Autodesk Fusion 360 part; units mm, degrees
note: some values were not read from the file. Chosen so that the rebuilt part matches the saved one: which bodies a step acts on; which pieces of a blend or face edit are solid. Set by a fixed rule: which sketch regions a step uses; the direction of a hole.
(part 2 of 2)
  constraint tangent L118 A111
  constraint tangent L136 A111
  constraint equal A56 A111
  constraint tangent L131 A112
  constraint tangent L136 A112
  constraint equal A56 A112
  constraint tangent L124 A113
  constraint tangent L133 A113
  constraint equal A56 A113
  constraint tangent L117 A114
  constraint tangent L124 A114
  constraint equal A56 A114
  constraint tangent L139 A115
  constraint tangent L141 A115
  constraint equal A56 A115
  constraint tangent L141 A116
  constraint tangent L142 A116
  constraint equal A56 A116
  constraint tangent L142 A117
  constraint tangent L148 A117
  constraint equal A56 A117
  constraint tangent A115 A118
  constraint tangent L141 A118
  constraint equal A56 A118
  constraint tangent L139 A119
  constraint tangent L148 A119
  constraint equal A56 A119
  constraint tangent L147 A120
  constraint tangent L152 A120
  constraint equal A56 A120
  constraint tangent L150 A121
  constraint tangent L152 A121
  constraint equal A56 A121
  constraint tangent L144 A122
  constraint tangent L147 A122
  constraint equal A56 A122
  constraint tangent L144 A123
  constraint tangent L150 A123
  constraint equal A56 A123
  constraint tangent L140 A124
  constraint tangent L151 A124
  constraint equal A56 A124
  constraint tangent L145 A125
  constraint tangent L151 A125
  constraint equal A56 A125
  constraint tangent L140 A126
  constraint tangent L149 A126
  constraint equal A56 A126
  constraint tangent L145 A127
  constraint tangent L149 A127
  constraint equal A56 A127
  constraint tangent L271 A128
  constraint tangent L272 A128
  constraint equal A56 A128
  constraint coincident P21 L272
  constraint coincident P21 L273
  constraint tangent L272 A129
  constraint tangent L273 A129
  constraint equal A56 A129
  constraint coincident P19 L270
  constraint coincident P19 L273
  constraint tangent L270 A130
  constraint tangent L273 A130
  constraint equal A56 A130
  constraint coincident P20 L270
  constraint coincident P20 L271
  constraint tangent L270 A131
  constraint tangent L271 A131
  constraint equal A56 A131
  constraint coincident L128.end L130
  constraint coincident L128.end L112
  constraint tangent L130 A132
  constraint tangent L112 A132
  constraint coincident P18 L267
  constraint coincident P18 L268
  constraint tangent L267 A133
  constraint tangent L268 A133
  constraint tangent L266 A134
  constraint tangent L267 A134
  constraint equal A133 A134
  constraint tangent L265 A135
  constraint tangent L266 A135
  constraint equal A133 A135
  constraint coincident P17 L265
  constraint coincident P17 L268
  constraint tangent L265 A136
  constraint tangent L268 A136
  constraint equal A133 A136
  constraint tangent L249 A137
  constraint tangent L259 A137
  constraint equal A133 A137
  constraint tangent L253 A138
  constraint tangent L259 A138
  constraint equal A133 A138
  constraint tangent L253 A139
  constraint tangent L254 A139
  constraint equal A133 A139
  constraint tangent L249 A140
  constraint tangent L254 A140
  constraint equal A133 A140
  constraint tangent L255 A141
  constraint tangent L260 A141
  constraint equal A133 A141
  constraint tangent L257 A142
  constraint tangent L260 A142
  constraint equal A133 A142
  constraint tangent L251 A143
  constraint tangent L257 A143
  constraint equal A133 A143
  constraint tangent L251 A144
  constraint tangent L255 A144
  constraint equal A133 A144
  constraint tangent L256 A145
  constraint tangent L263 A145
  constraint equal A133 A145
  constraint tangent L263 A146
  constraint tangent L264 A146
  constraint equal A133 A146
  constraint tangent L252 A147
  constraint tangent L264 A147
  constraint equal A133 A147
  constraint tangent L252 A148
  constraint tangent L256 A148
  constraint equal A133 A148
  constraint tangent L250 A149
  constraint tangent L261 A149
  constraint equal A133 A149
  constraint tangent L261 A150
  constraint tangent L262 A150
  constraint equal A133 A150
  constraint tangent L250 A151
  constraint tangent L258 A151
  constraint equal A133 A151
  constraint tangent L258 A152
  constraint tangent L262 A152
  constraint equal A133 A152
  constraint tangent L242 A153
  constraint tangent L246 A153
  constraint equal A133 A153
  constraint tangent L229 A154
  constraint tangent L242 A154
  constraint equal A133 A154
  constraint tangent L229 A155
  constraint tangent L245 A155
  constraint equal A133 A155
  constraint tangent L245 A156
  constraint tangent L246 A156
  constraint equal A133 A156
  constraint tangent L235 A157
  constraint tangent L248 A157
  constraint equal A133 A157
  constraint tangent L248 A158
  constraint tangent L247 A158
  constraint equal A133 A158
  constraint tangent L240 A159
  constraint tangent L247 A159
  constraint equal A133 A159
  constraint tangent L235 A160
  constraint tangent L240 A160
  constraint equal A133 A160
  constraint tangent L241 A161
  constraint tangent L244 A161
  constraint equal A133 A161
  constraint tangent L234 A162
  constraint tangent L241 A162
  constraint equal A133 A162
  constraint tangent L238 A163
  constraint tangent L244 A163
  constraint equal A133 A163
  constraint tangent L234 A164
  constraint tangent L238 A164
  constraint equal A133 A164
  constraint tangent L236 A165
  constraint tangent L243 A165
  constraint equal A133 A165
  constraint tangent L236 A166
  constraint tangent L237 A166
  constraint equal A133 A166
  constraint tangent L225 A167
  constraint tangent L243 A167
  constraint equal A133 A167
  constraint tangent L225 A168
  constraint tangent L237 A168
  constraint equal A133 A168
  constraint tangent L201 A169
  constraint tangent L219 A169
  constraint equal A133 A169
  constraint tangent L201 A170
  constraint tangent L213 A170
  constraint equal A133 A170
  constraint tangent L212 A171
  constraint tangent L219 A171
  constraint equal A133 A171
  constraint tangent L212 A172
  constraint tangent L213 A172
  constraint equal A133 A172
  constraint tangent L214 A173
  constraint tangent L220 A173
  constraint equal A133 A173
  constraint tangent L210 A174
  constraint tangent L214 A174
  constraint equal A133 A174
  constraint tangent L217 A175
  constraint tangent L220 A175
  constraint equal A133 A175
  constraint tangent L210 A176
  constraint tangent L217 A176
  constraint equal A133 A176
  constraint tangent L216 A177
  constraint tangent L223 A177
  constraint equal A133 A177
  constraint tangent L211 A178
  constraint tangent L216 A178
  constraint equal A133 A178
  constraint tangent L223 A179
  constraint tangent L224 A179
  constraint equal A133 A179
  constraint tangent L211 A180
  constraint tangent L224 A180
  constraint equal A133 A180
  constraint tangent L205 A181
  constraint tangent L221 A181
  constraint equal A133 A181
  constraint tangent L221 A182
  constraint tangent L222 A182
  constraint equal A133 A182
  constraint tangent L205 A183
  constraint tangent L218 A183
  constraint equal A133 A183
  constraint tangent L218 A184
  constraint tangent L222 A184
  constraint equal A133 A184
  constraint tangent L227 A185
  constraint tangent L230 A185
  constraint equal A133 A185
  constraint tangent L227 A186
  constraint tangent L228 A186
  constraint equal A133 A186
  constraint tangent L230 A187
  constraint tangent L231 A187
  constraint equal A133 A187
  constraint tangent L228 A188
  constraint tangent L231 A188
  constraint equal A133 A188
  constraint tangent L226 A189
  constraint tangent L233 A189
  constraint equal A133 A189
  constraint tangent L233 A190
  constraint tangent L239 A190
  constraint equal A133 A190
  constraint tangent L226 A191
  constraint tangent L232 A191
  constraint equal A133 A191
  constraint tangent L232 A192
  constraint tangent L239 A192
  constraint equal A133 A192
  constraint tangent L203 A193
  constraint tangent L206 A193
  constraint equal A133 A193
  constraint tangent L206 A194
  constraint tangent L207 A194
  constraint equal A133 A194
  constraint tangent L204 A195
  constraint tangent L207 A195
  constraint equal A133 A195
  constraint tangent L203 A196
  constraint tangent L204 A196
  constraint equal A133 A196
  constraint tangent L202 A197
  constraint tangent L209 A197
  constraint equal A133 A197
  constraint tangent L202 A198
  constraint tangent L208 A198
  constraint equal A133 A198
  constraint tangent L208 A199
  constraint tangent L215 A199
  constraint equal A133 A199
  constraint tangent L209 A200
  constraint tangent L215 A200
  constraint equal A133 A200
  constraint tangent L181 A201
  constraint tangent L190 A201
  constraint equal A133 A201
  constraint tangent L190 A202
  constraint tangent L197 A202
  constraint equal A133 A202
  constraint tangent L178 A203
  constraint tangent L181 A203
  constraint equal A133 A203
  constraint tangent L178 A204
  constraint tangent L197 A204
  constraint equal A133 A204
  constraint tangent L177 A205
  constraint tangent L198 A205
  constraint equal A133 A205
  constraint tangent L180 A206
  constraint tangent L198 A206
  constraint equal A133 A206
  constraint tangent L180 A207
  constraint tangent L193 A207
  constraint equal A133 A207
  constraint tangent L177 A208
  constraint tangent L193 A208
  constraint equal A133 A208
  constraint tangent L192 A209
  constraint tangent L196 A209
  constraint equal A133 A209
  constraint tangent L179 A210
  constraint tangent L192 A210
  constraint equal A133 A210
  constraint tangent L179 A211
  constraint tangent L199 A211
  constraint equal A133 A211
  constraint tangent L196 A212
  constraint tangent L199 A212
  constraint equal A133 A212
  constraint tangent L185 A213
  constraint tangent L194 A213
  constraint equal A133 A213
  constraint tangent L185 A214
  constraint tangent L186 A214
  constraint equal A133 A214
  constraint tangent L186 A215
  constraint tangent L188 A215
  constraint equal A133 A215
  constraint tangent L188 A216
  constraint tangent L194 A216
  constraint equal A133 A216
  constraint tangent L166 A217
  constraint tangent L168 A217
  constraint equal A133 A217
  constraint tangent L167 A218
  constraint tangent L168 A218
  constraint equal A133 A218
  constraint tangent L165 A219
  constraint tangent L167 A219
  constraint equal A133 A219
  constraint tangent L165 A220
  constraint tangent L166 A220
  constraint equal A133 A220
  constraint tangent L163 A221
  constraint tangent L164 A221
  constraint equal A133 A221
  constraint tangent L161 A222
  constraint tangent L163 A222
  constraint equal A133 A222
  constraint tangent L162 A223
  constraint tangent L164 A223
  constraint equal A133 A223
  constraint tangent L161 A224
  constraint tangent L162 A224
  constraint equal A133 A224
  constraint tangent L159 A225
  constraint tangent L160 A225
  constraint equal A133 A225
  constraint tangent L157 A226
  constraint tangent L159 A226
  constraint equal A133 A226
  constraint tangent L158 A227
  constraint tangent L160 A227
  constraint equal A133 A227
  constraint tangent L157 A228
  constraint tangent L158 A228
  constraint equal A133 A228
  constraint tangent L154 A229
  constraint tangent L155 A229
  constraint equal A133 A229
  constraint tangent L153 A230
  constraint tangent L154 A230
  constraint equal A133 A230
  constraint tangent L155 A231
  constraint tangent L156 A231
  constraint equal A133 A231
  constraint tangent L153 A232
  constraint tangent L156 A232
  constraint equal A133 A232
  constraint tangent L170 A233
  constraint tangent L172 A233
  constraint equal A133 A233
  constraint tangent L171 A234
  constraint tangent L172 A234
  constraint equal A133 A234
  constraint tangent L169 A235
  constraint tangent L171 A235
  constraint equal A133 A235
  constraint tangent L169 A236
  constraint tangent L170 A236
  constraint equal A133 A236
  constraint tangent L173 A237
  constraint tangent L174 A237
  constraint equal A133 A237
  constraint tangent L174 A238
  constraint tangent L176 A238
  constraint equal A133 A238
  constraint tangent L175 A239
  constraint tangent L176 A239
  constraint equal A133 A239
  constraint tangent L173 A240
  constraint tangent L175 A240
  constraint equal A133 A240
  constraint tangent L184 A241
  constraint tangent L187 A241
  constraint equal A133 A241
  constraint tangent L182 A242
  constraint tangent L184 A242
  constraint equal A133 A242
  constraint tangent L182 A243
  constraint tangent L183 A243
  constraint equal A133 A243
  constraint tangent L183 A244
  constraint tangent L187 A244
  constraint equal A133 A244
  constraint tangent L189 A245
  constraint tangent L200 A245
  constraint equal A133 A245
  constraint tangent L189 A246
  constraint tangent L191 A246
  constraint equal A133 A246
  constraint tangent L191 A247
  constraint tangent L195 A247
  constraint equal A133 A247
  constraint tangent L195 A248
  constraint tangent L200 A248
  constraint equal A133 A248
  measures "d1" distance of L6.start L0.start
  measures "d2" distance of L0.start L0.end
  measures "d3" distance of L0.end L1.end
  measures "d7" distance of L4.end L5.end
  measures "d11" distance of L7.start L7.end
  measures "d12" distance of L7.end L8.end
  measures "d13" distance of L8.end L9.end
  measures "d15" distance of L10.end L11.end
  measures "d18" distance of L12.end L13.end
  measures "d87" distance of P17 P18
  measures "d90" distance of L13.end L269.end
  measures "d92" distance of P19 P21
  measures "d93" distance of P19 P20
  measures "d94" radius of A0
  measures "d95" radius of A16
  measures "d96" radius of A54
  measures "d97" radius of A55
  measures "d98" radius of A56
  measures "d99" radius of A132
  measures "d100" radius of A133
  measures "d105" distance of L11.end P22
extrude "Extrude1" add sketch "Sketch1" along normal blind 4 contours L0 L1 L2 L3 L4 L5 L6 L15 | L7 L8 L9 L10 L11 L12 L13 L14 L32 L269 | L16 L17 L18 L19 L20 L21 L22 L23 A8 A9 A10 A11 A12 A13 A14 A15 | L24 L25 L26 L27 L28 L29 L30 L31 A0 A1 A2 A3 A4 A5 A6 A7 makes body 1 at (38.1433, 0, -12.1134) makes body 2 at (-23.9522, 0, -12.611)
extrude "Extrude2" add sketch "Sketch1" against normal blind 1 contours L16 L17 L18 L19 L20 L21 L22 L23 A8 A9 A10 A11 A12 A13 A14 A15 | L24 L25 L26 L27 L28 L29 L30 L31 A0 A1 A2 A3 A4 A5 A6 A7 bodies 1 2
hole "Hole1" at (-123.1355, 0, 35.5) at (-18.6355, 0, 47) at (-125.6355, 0, 54.5) at (-9.1355, 0, 54.5) at (-9.1355, 0, -49) at (-161.6355, 0, -49) at (-161.6355, 0, 36.5) at (-155.1355, 0, -42) at (-15.3855, 0, -43.25) at (29.5, 0, -43) at (23.0255, 0, -48.5253) at (170.75, 0, -42) at (177.25, 0, -48.5) at (177.25, 0, 37) at (140.75, 0, 55) at (140.2499, 0, 35.0254) at (22, 0, 55) at (31.9999, 0, 47.1754) direction (0, 1, 0) diameter 2.1 end through all bodies 2 1
move_body "Move1" bodies 1 2 to x (1, 0, 0) y (0, 1, 0) z (0, 0, 1) at (0, 0, -140)
extrude "Extrude3" add sketch "Sketch1" along normal blind 8 separate body contours L0 L1 L2 L3 L4 L5 L6 L15 | L7 L8 L9 L10 L11 L12 L13 L14 L32 L269 | L16 L17 L18 L19 L20 L21 L22 L23 A8 A9 A10 A11 A12 A13 A14 A15 | L24 L25 L26 L27 L28 L29 L30 L31 A0 A1 A2 A3 A4 A5 A6 A7 | L34 L35 L36 L37 L38 A16 A17 A18 A54 | L39 L40 L41 L42 A19 A20 A21 A22 | L43 L44 L45 L46 A23 A24 A25 A26 | L47 L48 L49 L50 A27 A28 A29 A30 | L51 L52 L53 L54 A46 A47 A48 A49 | L55 L56 L57 L58 A84 A85 A86 A87 | L59 L64 L81 L84 A80 A81 A82 A83 | L60 L63 L73 L74 A39 A40 A41 A42 | L61 L62 L70 L71 L75 A43 A44 A45 A55 | L65 L66 L76 L79 A35 A36 A37 A38 | L67 L68 L78 L80 A31 A32 A33 A34 | L72 L77 L82 L83 A50 A51 A52 A53 | L85 L98 L104 L109 A60 A61 A62 A63 | L86 L95 L100 L101 A72 A73 A74 A75 | L87 L88 L96 L97 A68 A69 A70 A71 | L89 L90 L93 L94 A76 A77 A78 A79 | L91 L92 L99 L106 L110 A56 A57 A58 A59 | L102 L103 L105 L107 A64 A65 A66 A67 | L111 L113 L114 L132 A91 A92 A93 A94 | L112 L116 L128 L129 L130 A88 A89 A90 A132 | L115 L119 L121 L126 A99 A100 A101 A102 | L117 L124 L127 L133 A103 A104 A113 A114 | L118 L123 L131 L136 A105 A106 A111 A112 | L120 L125 L134 L135 A107 A108 A109 A110 | L137 L138 L143 L146 A95 A96 A97 A98 | L139 L141 L142 L148 A115 A116 A117 A118 A119 | L140 L145 L149 L151 A124 A125 A126 A127 | L144 L147 L150 L152 A120 A121 A122 A123 | L153 L154 L155 L156 A229 A230 A231 A232 | L157 L158 L159 L160 A225 A226 A227 A228 | L161 L162 L163 L164 A221 A222 A223 A224 | L165 L166 L167 L168 A217 A218 A219 A220 | L169 L170 L171 L172 A233 A234 A235 A236 | L173 L174 L175 L176 A237 A238 A239 A240 | L177 L180 L193 L198 A205 A206 A207 A208 | L178 L181 L190 L197 A201 A202 A203 A204 | L179 L192 L196 L199 A209 A210 A211 A212 | L182 L183 L184 L187 A241 A242 A243 A244 | L185 L186 L188 L194 A213 A214 A215 A216 | L189 L191 L195 L200 A245 A246 A247 A248 | L201 L212 L213 L219 A169 A170 A171 A172 | L202 L208 L209 L215 A197 A198 A199 A200 | L203 L204 L206 L207 A193 A194 A195 A196 | L205 L218 L221 L222 A181 A182 A183 A184 | L210 L214 L217 L220 A173 A174 A175 A176 | L211 L216 L223 L224 A177 A178 A179 A180 | L225 L236 L237 L243 A165 A166 A167 A168 | L226 L232 L233 L239 A189 A190 A191 A192 | L227 L228 L230 L231 A185 A186 A187 A188 | L229 L242 L245 L246 A153 A154 A155 A156 | L234 L238 L241 L244 A161 A162 A163 A164 | L235 L240 L247 L248 A157 A158 A159 A160 | L249 L253 L254 L259 A137 A138 A139 A140 | L250 L258 L261 L262 A149 A150 A151 A152 | L251 L255 L257 L260 A141 A142 A143 A144 | L252 L256 L263 L264 A145 A146 A147 A148 | L265 L266 L267 L268 A133 A134 A135 A136 | L270 L271 L272 L273 A128 A129 A130 A131 makes body 3 at (-99.9688, 0, -18.744) makes body 4 at (114.8434, 0, -18.244)
extrude "Extrude4" add sketch "Sketch1" along normal blind 13 separate body contours L16 L17 L18 L19 L20 L21 L22 L23 A8 A9 A10 A11 A12 A13 A14 A15 | L24 L25 L26 L27 L28 L29 L30 L31 A0 A1 A2 A3 A4 A5 A6 A7 makes body 5 at (-109.9688, 0, -49.8333) makes body 6 at (125.0101, 0, -49.3333)
combine "Combine1" operation add target body 3 tool bodies 5
combine "Combine2" operation add target body 6 tool bodies 4
sketch "Sketch2" plane through (0, 0, 0) normal (0, 1, 0) x (1, 0, 0)
  line L0 (-145, 32.4457) -> (-45, 32.4457)
  line L1 (-45, 32.4457) -> (-45, -27.5543)
  line L2 (-45, -27.5543) -> (-145, -27.5543)
  line L3 (-145, -27.5543) -> (-145, 32.4457)
  line L4 (60, 32.4457) -> (160, 32.4457)
  line L5 (160, -27.5543) -> (60, -27.5543)
  line L6 (160, 32.4457) -> (160, -27.5543)
  line L7 (60, -27.5543) -> (60, 32.4457)
  line L8 (-35, 40) -> (-15, 40)
  line L9 (-15, 40) -> (-15, 10)
  line L10 (-15, 10) -> (-35, 10)
  line L11 (-35, 10) -> (-35, 40)
  circle A0 centre (-30, 17.5) radius 2
  circle A1 centre (-20, 17.5) radius 2
  circle A2 centre (-20, 32.5) radius 2
  circle A3 centre (-30, 32.5) radius 2
  line L12 (-45.5, 25) -> (-34.5, 25)
  line L13 (-34.5, 25) -> (-34.5, 22)
  line L14 (-34.5, 22) -> (-45.5, 22)
  line L15 (-45.5, 22) -> (-45.5, 25)
  line L16 (60.5, 25) -> (49.5, 25)
  line L17 (49.5, 22) -> (60.5, 22)
  line L18 (49.5, 25) -> (49.5, 22)
  line L19 (50, 10) -> (50, 40)
  line L20 (60.5, 22) -> (60.5, 25)
  circle A4 centre (45, 32.5) radius 2
  circle A5 centre (35, 32.5) radius 2
  circle A6 centre (35, 17.5) radius 2
  circle A7 centre (45, 17.5) radius 2
  line L21 (30, 40) -> (30, 10)
  line L22 (30, 10) -> (50, 10)
  line L23 (50, 40) -> (30, 40)
  line L24 (-30, -5) -> (-32.5, -9.3301)
  line L25 (-32.5, -9.3301) -> (-30, -13.6603)
  line L26 (-30, -13.6603) -> (-25, -13.6603)
  line L27 (-25, -13.6603) -> (-22.5, -9.3301)
  line L28 (-22.5, -9.3301) -> (-25, -5)
  line L29 (-25, -5) -> (-30, -5)
  line L30 (-16, -8.6603) -> (-13.5, -4.3301)
  line L31 (-21, -8.6603) -> (-16, -8.6603)
  line L32 (-16, 0) -> (-21, 0)
  line L33 (-13.5, -4.3301) -> (-16, 0)
  line L34 (-23.5, -4.3301) -> (-21, -8.6603)
  line L35 (-21, 0) -> (-23.5, -4.3301)
  line L36 (-16, -18.6603) -> (-13.5, -14.3301)
  line L37 (-21, -18.6603) -> (-16, -18.6603)
  line L38 (-16, -10) -> (-21, -10)
  line L39 (-13.5, -14.3301) -> (-16, -10)
  line L40 (-23.5, -14.3301) -> (-21, -18.6603)
  line L41 (-21, -10) -> (-23.5, -14.3301)
  line L42 (-25, -3.6603) -> (-22.5, 0.6699)
  line L43 (-30, -3.6603) -> (-25, -3.6603)
  line L44 (-25, 5) -> (-30, 5)
  line L45 (-22.5, 0.6699) -> (-25, 5)
  line L46 (-32.5, 0.6699) -> (-30, -3.6603)
  line L47 (-30, 5) -> (-32.5, 0.6699)
  line L48 (-25, -23.6603) -> (-22.5, -19.3301)
  line L49 (-30, -23.6603) -> (-25, -23.6603)
  line L50 (-25, -15) -> (-30, -15)
  line L51 (-22.5, -19.3301) -> (-25, -15)
  line L52 (-32.5, -19.3301) -> (-30, -23.6603)
  line L53 (-30, -15) -> (-32.5, -19.3301)
  line L54 (-16, 1.3397) -> (-13.5, 5.6699)
  line L55 (-21, 1.3397) -> (-16, 1.3397)
  line L56 (-16, 10) -> (-21, 10)
  line L57 (-13.5, 5.6699) -> (-16, 10)
  line L58 (-23.5, 5.6699) -> (-21, 1.3397)
  line L59 (-21, 10) -> (-23.5, 5.6699)
  line L60 (-34, -33.6603) -> (-31.5, -29.3301)
  line L61 (-39, -33.6603) -> (-34, -33.6603)
  line L62 (-34, -25) -> (-39, -25)
  line L63 (-31.5, -29.3301) -> (-34, -25)
  line L64 (-41.5, -29.3301) -> (-39, -33.6603)
  line L65 (-39, -25) -> (-41.5, -29.3301)
  line L66 (-25, -13.6603) -> (-22.5, -9.3301)
  line L67 (-30, -13.6603) -> (-25, -13.6603)
  line L68 (-25, -5) -> (-30, -5)
  line L69 (-22.5, -9.3301) -> (-25, -5)
  line L70 (-32.5, -9.3301) -> (-30, -13.6603)
  line L71 (-30, -5) -> (-32.5, -9.3301)
  line L72 (39, -14.3301) -> (36.5, -18.6603)
  line L73 (39, 5.6699) -> (36.5, 1.3397)
  line L74 (36.5, -18.6603) -> (31.5, -18.6603)
  line L75 (40.5, -5) -> (45.5, -5)
  line L76 (45.5, 5) -> (48, 0.6699)
  line L77 (36.5, 10) -> (39, 5.6699)
  line L78 (36.5, 0) -> (39, -4.3301)
  line L79 (31.5, -8.6603) -> (29, -4.3301)
  line L80 (29, 5.6699) -> (31.5, 10)
  line L81 (38, 0.6699) -> (40.5, 5)
  line L82 (38, -9.3301) -> (40.5, -5)
  line L83 (45.5, -5) -> (48, -9.3301)
  line L84 (29, -4.3301) -> (31.5, 0)
  line L85 (40.5, -23.6603) -> (38, -19.3301)
  line L86 (48, -9.3301) -> (45.5, -13.6603)
  line L87 (29, -14.3301) -> (31.5, -10)
  line L88 (48, -19.3301) -> (45.5, -23.6603)
  line L89 (48, -9.3301) -> (45.5, -13.6603)
  line L90 (45.5, -13.6603) -> (40.5, -13.6603)
  line L91 (40.5, -13.6603) -> (38, -9.3301)
  line L92 (40.5, -3.6603) -> (38, 0.6699)
  line L93 (40.5, 5) -> (45.5, 5)
  line L94 (31.5, 1.3397) -> (29, 5.6699)
  line L95 (36.5, 1.3397) -> (31.5, 1.3397)
  line L96 (31.5, 0) -> (36.5, 0)
  line L97 (45.5, -3.6603) -> (40.5, -3.6603)
  line L98 (48, 0.6699) -> (45.5, -3.6603)
  line L99 (40.5, -5) -> (45.5, -5)
  line L100 (31.5, 10) -> (36.5, 10)
  line L101 (39, -4.3301) -> (36.5, -8.6603)
  line L102 (38, -9.3301) -> (40.5, -5)
  line L103 (49.5, -25) -> (54.5, -25)
  line L104 (30.5, 10) -> (50.5, 10)
  line L105 (45.5, -5) -> (48, -9.3301)
  line L106 (36.5, -10) -> (39, -14.3301)
  line L107 (31.5, -18.6603) -> (29, -14.3301)
  line L108 (40.5, -15) -> (45.5, -15)
  line L109 (45.5, -23.6603) -> (40.5, -23.6603)
  line L110 (38, -19.3301) -> (40.5, -15)
  line L111 (45.5, -13.6603) -> (40.5, -13.6603)
  line L112 (31.5, -10) -> (36.5, -10)
  line L113 (40.5, -13.6603) -> (38, -9.3301)
  line L114 (36.5, -8.6603) -> (31.5, -8.6603)
  line L115 (45.5, -15) -> (48, -19.3301)
  line L116 (57, -29.3301) -> (54.5, -33.6603)
  line L117 (47, -29.3301) -> (49.5, -25)
  line L118 (54.5, -33.6603) -> (49.5, -33.6603)
  line L119 (49.5, -33.6603) -> (47, -29.3301)
  line L120 (54.5, -25) -> (57, -29.3301)
  line L121 (-2.7, 45) -> (0.1, 45)
  line L122 (0.4, 44.7) -> (0.4, 36.1)
  line L123 (0.1, 35.8) -> (-2.7, 35.8)
  line L124 (-3, 36.1) -> (-3, 44.7)
  arc A8 (0.4, 44.7) -> (0.1, 45) centre (0.1, 44.7) ccw
  arc A9 (-2.7, 45) -> (-3, 44.7) centre (-2.7, 44.7) ccw
  arc A10 (-3, 36.1) -> (-2.7, 35.8) centre (-2.7, 36.1) ccw
  arc A11 (0.1, 35.8) -> (0.4, 36.1) centre (0.1, 36.1) ccw
  line L125 (-3.5, 34) -> (2.7, 34)
  line L126 (3, 33.7) -> (3, 21.5)
  line L127 (2.7, 21.2) -> (-3.5, 21.2)
  line L128 (-3.8, 21.5) -> (-3.8, 33.7)
  arc A12 (-3.5, 34) -> (-3.8, 33.7) centre (-3.5, 33.7) ccw
  arc A13 (3, 33.7) -> (2.7, 34) centre (2.7, 33.7) ccw
  arc A14 (2.7, 21.2) -> (3, 21.5) centre (2.7, 21.5) ccw
  arc A15 (-3.8, 21.5) -> (-3.5, 21.2) centre (-3.5, 21.5) ccw
  point P0 (-27.5, -9.3301)
  point P1 (-18.5, -4.3301)
  point P2 (-18.5, -14.3301)
  point P3 (-27.5, 0.6699)
  point P4 (-27.5, -19.3301)
  point P5 (-18.5, 5.6699)
  point P6 (-36.5, -29.3301)
  point P7 (-27.5, -9.3301)
  point P8 (15.5, 0)
  point P9 (43, -9.3301)
  point P10 (52, -29.3301)
  point P11 (34, -4.3301)
  point P12 (43, -9.3301)
  point P13 (34, -14.3301)
  point P14 (43, -19.3301)
  point P15 (43, 0.6699)
  point P16 (34, 5.6699)
  point P17 (-3, 45)
  point P18 (0.4, 45)
  point P19 (-3, 35.8)
  point P20 (-3.8, 34)
  point P21 (3, 21.2)
  point P22 (-3.8, 21.2)
  dimension "d138" = 3.4
  dimension "d139" = 9.2
  dimension "d140" = 0.3
  dimension "d141" = 6.8
  dimension "d142" = 12.8
  dimension "d143" = 0.3
  constraint horizontal L0
  constraint vertical L1
  constraint horizontal L2
  constraint vertical L3
  constraint horizontal L4
  constraint vertical L6
  constraint horizontal L5
  constraint vertical L7
  constraint horizontal L8
  constraint vertical L9
  constraint horizontal L10
  constraint vertical L11
  constraint horizontal L12
  constraint perpendicular L12 L13
  constraint perpendicular L1 L14
  constraint perpendicular L12 L15
  constraint perpendicular L16 L18
  constraint perpendicular L16 L20
  constraint horizontal L121
  constraint vertical L122
  constraint horizontal L123
  constraint vertical L124
  constraint coincident P18 L121
  constraint coincident P18 L122
  constraint tangent L121 A8
  constraint tangent L122 A8
  constraint coincident P17 L121
  constraint coincident P17 L124
  constraint tangent L121 A9
  constraint tangent L124 A9
  constraint equal A8 A9
  constraint coincident P19 L123
  constraint coincident P19 L124
  constraint tangent L123 A10
  constraint tangent L124 A10
  constraint equal A8 A10
  constraint tangent L122 A11
  constraint tangent L123 A11
  constraint equal A8 A11
  constraint horizontal L125
  constraint vertical L126
  constraint horizontal L127
  constraint vertical L128
  constraint coincident P20 L125
  constraint coincident P20 L128
  constraint tangent L125 A12
  constraint tangent L128 A12
  constraint tangent L125 A13
  constraint tangent L126 A13
  constraint equal A12 A13
  constraint coincident P21 L126
  constraint coincident P21 L127
  constraint tangent L126 A14
  constraint tangent L127 A14
  constraint equal A12 A14
  constraint coincident P22 L127
  constraint coincident P22 L128
  constraint tangent L127 A15
  constraint tangent L128 A15
  constraint equal A12 A15
  measures "d138" distance of P17 P18
  measures "d139" distance of P17 P19
  measures "d140" radius of A8
  measures "d141" distance of P21 P22
  measures "d142" distance of P20 P22
  measures "d143" radius of A12
extrude "Extrude5" add sketch "Sketch2" along normal blind 4.5 separate body contours L0 L1 L2 L3 L12 L14 L15 | L1 L12 L14 L15 | L4 L5 L6 L7 L16 L17 L20 | L7 L16 L17 L20 makes body 7 at (-111.6667, 0, -12.4457) makes body 8 at (93.3333, 0, -12.4457)
move_body "Move2" bodies 7 8 to x (1, 0, 0) y (0, 1, 0) z (0, 0, 1) at (0, 4, 0)
combine "Combine3" operation cut target body 3 tool bodies 7
combine "Combine4" operation cut target body 6 tool bodies 8
chamfer "Chamfer1" distance 2 angle 45 8 edges at (110, 8, -32.4457) (110, 4, -32.4457) (60, 8, -2.4457) (160, 8, -2.4457) (160, 4, -2.4457) (110, 8, 27.5543) (110, 4, 27.5543) (60, 4, -2.4457) on bodies 6
chamfer "Chamfer2" distance 2 angle 45 8 edges at (-145, 4, -2.4457) (-145, 8, -2.4457) (-95, 8, -32.4457) (-95, 4, -32.4457) (-95, 8, 27.5543) (-45, 8, -2.4457) (-45, 4, -2.4457) (-95, 4, 27.5543) on bodies 3
extrude "Extrude6" add sketch "Sketch2" along normal blind 3 separate body contours L7 L16 L17 L20 | L7 L16 L17 L19 | L16 L17 L18 L19 | L16 L17 L18 L19 L21 L22 L23 L100 L104 | A4 | A5 | A6 | A7 makes body 9
move_body "Move3" bodies 9 to x (1, 0, 0) y (0, 1, 0) z (0, 0, 1) at (0, 5, -6)
combine "Combine5" operation cut target body 6 tool bodies 9
chamfer "Chamfer3" distance 0.5 angle 45 16 edges at (54, 8, -28) (54, 8, -31) (59.25, 6.75, -28) (59.25, 6.75, -31) (50, 6.5, -28) (50, 5, -22) (50, 8, -22) (50, 6.5, -31) (50, 8, -38.5) (50, 5, -38.5) (40, 5, -16) (40, 8, -16) (30, 8, -31) (30, 5, -31) (30, 6.5, -16) (50, 6.5, -16) on bodies 6
extrude "Extrude7" add sketch "Sketch2" along normal blind 3 separate body contours L1 L11 L12 L14 | L1 L12 L14 L15 | L11 L12 L13 L14 | L8 L9 L10 L11 L12 L13 L14 L56 | A0 | A1 | A2 | A3 makes body 10
move_body "Move4" bodies 10 to x (1, 0, 0) y (0, 1, 0) z (0, 0, 1) at (0, 0, -6.5)
move_body "Move5" bodies 10 to x (1, 0, 0) y (0, 1, 0) z (0, 0, 1) at (0, 5, 0)
combine "Combine6" operation cut target body 3 tool bodies 10
chamfer "Chamfer4" distance 0.5 angle 45 14 edges at (-15, 8, -31.5) (-15, 5, -31.5) (-35, 8, -39) (-39, 8, -31.5) (-39, 8, -28.5) (-35, 8, -22.5) (-25, 8, -16.5) (-35, 5, -22.5) (-25, 5, -16.5) (-35, 6.5, -16.5) (-35, 6.5, -28.5) (-35, 6.5, -31.5) (-35, 5, -39) (-15, 6.5, -16.5) on bodies 3
chamfer "Chamfer5" distance 0.5 angle 45 2 edges at (-35, 6.5, -46.5) (-45.5, 5.5, -30) on bodies 3
chamfer "Chamfer6" distance 0.5 angle 45 1 edges at (60.5, 5.5, -29.5) on bodies 6
chamfer "Chamfer7" distance 0.5 angle 45 8 edges at (25, 13, 3.25) (100.125, 13, -46) (81.375, 13, 52.5) (138.25, 13, 47.25) (144, 13, 42) (149.75, 13, 38.25) (162.25, 13, 34.5) (174.75, 13, -5.75) on bodies 6
chamfer "Chamfer8" distance 0.5 angle 45 8 edges at (-159.1355, 13, -6.25) (-85.3855, 13, -46.5) (-146.8855, 13, 34) (-134.6355, 13, 37.75) (-128.8855, 13, 41.5) (-123.1355, 13, 46.75) (-67.3855, 13, 52) (-11.6355, 13, 2.75) on bodies 3
extrude "Extrude8" add sketch "Sketch2" along normal blind 2 separate body contours A0 | A1 | A2 | A3 | A4 | A5 | A6 | A7 makes body 11 at (35.5417, 1.3333, -19.4252) makes body 12 at (-18.0025, 1.3333, -17.4003) makes body 13 at (-21.9382, 0.6667, -32.9935) makes body 14 at (45.5417, 1.3333, -19.4252) makes body 15 at (35.0499, 1.3333, -34.4994) makes body 16 at (-28.0025, 1.3333, -17.4003) makes body 17 at (-31.9901, 1.3333, -32.3009) makes body 18 at (44.363, 1.3333, -30.6041)
move_body "Move6" bodies 12 13 16 17 to x (1, 0, 0) y (0, 1, 0) z (0, 0, 1) at (0, 4, -6)
combine "Combine7" operation cut target body 3 tool bodies 16 17 13 12
chamfer "Chamfer9" distance 0.2 angle 45 4 edges at (-21.8647, 5, -39.2232) (-31.8647, 5, -39.2232) (-31.8647, 5, -24.2232) (-21.8647, 5, -24.2232) on bodies 3
move_body "Move7" bodies 11 14 15 18 to x (1, 0, 0) y (0, 1, 0) z (0, 0, 1) at (0, 4, -6)
combine "Combine8" operation cut target body 6 tool bodies 14 18 15 11
chamfer "Chamfer10" distance 0.2 angle 45 4 edges at (36.8647, 5, -37.7768) (46.8647, 5, -37.7768) (46.8647, 5, -22.7768) (36.8647, 5, -22.7768) on bodies 6
extrude "Extrude9" add sketch "Sketch2" along normal blind 2.5 separate body contours L10 L54 L55 L56 L57 L58 L59 | L22 L73 L77 L80 L94 L95 L100 L104 | L24 L25 L26 L27 L28 L29 L66 L67 L68 L69 L70 L71 | L30 L31 L32 L33 L34 L35 | L36 L37 L38 L39 L40 L41 | L42 L43 L44 L45 L46 L47 | L48 L49 L50 L51 L52 L53 | L60 L61 L62 L63 L64 L65 | L72 L74 L87 L106 L107 L112 | L75 L82 L83 L86 L89 L90 L91 L99 L102 L105 L111 L113 | L76 L81 L92 L93 L97 L98 | L78 L79 L84 L96 L101 L114 | L85 L88 L108 L109 L110 L115 | L103 L116 L117 L118 L119 L120 makes body 19 at (34.8333, 0, 15.7735) makes body 20 at (35.6667, 0, -5.6699) makes body 21 at (-26.6667, 0, 10.7735) makes body 22 at (-17.6667, 0, -4.2265) makes body 23 at (-19.3333, 0, 15.7735) makes body 24 at (43.8333, 0, 0.7735) makes body 25 at (43.8333, 0, 17.8868) makes body 26 at (43.8333, 0, 10.7735) makes body 27 at (-37.3333, 0, 30.7735) makes body 28 at (-17.6667, 0, 5.7735) makes body 29 at (-26.6667, 0, 0.7735) makes body 30 at (-26.6667, 0, 17.8868) makes body 31 at (32.3333, 0, 4.3301) makes body 32 at (51.1667, 0, 30.7735)
move_body "Move8" bodies 19 20 21 22 32 31 25 29 23 26 27 28 30 24 to x (1, 0, 0) y (0, 1, 0) z (0, 0, 1) at (0, 7, 10)
combine "Combine9" operation cut target body 3 tool bodies 22 29 28 21 23 30 27
combine "Combine10" operation cut target body 6 tool bodies 24 20 31 26 19 25 32
hole "Hole2" at (-161.6355, 0, -49) at (-9.1355, 0, -49) at (23.0255, 0, -48.5253) at (177.25, 0, -48.5) at (177.25, 0, 37) at (152.75, 0, 45) at (140.75, 0, 55) at (22, 0, 55) at (-9.1355, 0, 54.5) at (-125.6355, 0, 54.5) at (-161.6355, 0, 36.5) direction (0, 1, 0) diameter 2.2 end through all counterbore diameter 3 counterbore depth 1.3 bodies 3 6
chamfer "Chamfer11" distance 0.7 angle 45 16 edges at (19.9999, 4, -136.7703) (20.048, 4, -83.093) (81.3597, 4, -82.5) (142.6642, 4, -83.0858) (143.25, 4, -87.75) (143.8358, 4, -92.4142) (149, 4, -93) (154.1642, 4, -93.5858) (154.75, 4, -96.75) (155.3358, 4, -99.9142) (167.25, 4, -100.5) (179.1642, 4, -101.0858) (179.75, 4, -145.75) (179.1642, 4, -190.4142) (100.1402, 4, -191) (21.1233, 4, -190.4214) on bodies 1
chamfer "Chamfer12" distance 0.7 angle 45 16 edges at (-6.6355, 4, -137.25) (-7.2212, 4, -190.9142) (-85.3855, 4, -191.5) (-163.5497, 4, -190.9142) (-164.1355, 4, -146.25) (-163.5497, 4, -101.5858) (-151.8855, 4, -101) (-140.2212, 4, -100.4142) (-139.6355, 4, -97.25) (-139.0497, 4, -94.0858) (-133.8855, 4, -93.5) (-128.7212, 4, -92.9142) (-128.1355, 4, -88.25) (-127.5497, 4, -83.5858) (-67.3855, 4, -83) (-7.2212, 4, -83.5858) on bodies 2
extrude "Extrude10" add sketch "Sketch2" along normal blind 9 separate body contours L121 L122 L123 L124 A8 A9 A10 A11 makes body 33
copy_body "CopyPasteBodies1" bodies 33 makes body 34
move_body "Move9" bodies 34 to x (0, -1, 0) y (0, 0, -1) z (1, 0, 0) at (15.5, 6, -45)
combine "Combine11" operation cut target body 3 tool bodies 34
chamfer "Chamfer13" distance 0.6 angle 45 8 edges at (-24.9, 5.6, -46.5) (-29.4121, 5.6879, -46.5) (-29.5, 7.3, -46.5) (-29.4121, 8.9121, -46.5) (-24.9, 9, -46.5) (-20.3879, 8.9121, -46.5) (-20.3, 7.3, -46.5) (-20.3879, 5.6879, -46.5) on bodies 3
move_body "Move10" bodies 33 to x (0, 1, 0) y (0, 0, -1) z (-1, 0, 0) at (-0.25, 8.5, -44)
combine "Combine12" operation cut target body 6 tool bodies 33
chamfer "Chamfer14" distance 1 angle 45 8 edges at (40.15, 5.5, -46) (35.6379, 5.5879, -46) (35.55, 7.2, -46) (35.6379, 8.8121, -46) (40.15, 8.9, -46) (44.6621, 8.8121, -46) (44.75, 7.2, -46) (44.6621, 5.5879, -46) on bodies 6
chamfer "Chamfer15" distance 0.5 angle 45 7 edges at (-29.8364, 5.2636, -46.5) (-19.9636, 5.2636, -46.5) (-19.7, 7.3, -46.5) (-19.9636, 9.3364, -46.5) (-24.9, 9.6, -46.5) (-29.8364, 9.3364, -46.5) (-30.1, 7.3, -46.5) on bodies 3
extrude "Extrude11" add sketch "Sketch2" along normal blind 20 separate body contours L125 L126 L127 L128 A12 A13 A14 A15 makes body 35
copy_body "CopyPasteBodies2" bodies 35 makes body 36
move_body "Move11" bodies 36 to x (0, 1, 0) y (0, 0, 1) z (1, 0, 0) at (-28.8, 7.8, -52)
combine "Combine13" operation cut target body 3 tool bodies 36
chamfer "Chamfer16" distance 0.5 angle 45 10 edges at (-50, 9.25, -46.5) (-62.8, 9.25, -46.5) (-62.7121, 10.7121, -46.5) (-56.4, 10.8, -46.5) (-50.0879, 10.7121, -46.5) (-50, 8, -40.4729) (-62.8, 8, -40.4729) (-62.8, 6.7771, -33.2229) (-50, 6.7771, -33.2229) (-56.4, 5.5543, -32) on bodies 3
chamfer "Chamfer17" distance 0.5 angle 45 5 edges at (-56.4, 11.3, -46.5) (-63.0657, 11.0657, -46.5) (-63.3, 9.25, -46.5) (-49.5, 9.25, -46.5) (-49.7343, 11.0657, -46.5) on bodies 3
chamfer "Chamfer18" distance 0.3 angle 45 1 edges at (-56.4, 5.2007, -31.6464) on bodies 3
move_body "Move12" bodies 35 to x (0, 1, 0) y (0, 0, 1) z (1, 0, 0) at (97.2, 7.8, -52)
combine "Combine14" operation cut target body 6 tool bodies 35
chamfer "Chamfer19" distance 1 angle 45 5 edges at (69.6, 10.8, -46) (75.9121, 10.7121, -46) (76, 9.25, -46) (63.2, 9.25, -46) (63.2879, 10.7121, -46) on bodies 6
chamfer "Chamfer20" distance 0.5 angle 45 5 edges at (63.2, 8, -40.7229) (63.2, 6.7771, -33.2229) (69.6, 5.5543, -32) (76, 6.7771, -33.2229) (76, 8, -40.7229) on bodies 6
chamfer "Chamfer21" distance 0.3 angle 45 1 edges at (69.6, 5.2007, -31.6464) on bodies 6
